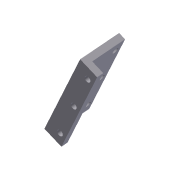
# Autodesk Inventor part: Trapezium
Saved by Autodesk Inventor 2011 (Build 150239000, 239)
## iProperties
Created: 2010-11-23
Part Number: Trapezium
Document SubType Name: Modeling
Designer: Milton
Density: 2.71 g/cm^3
Mass: 8.52062 g
Surface Area: 26.6037 cm^2
Volume: 3.14414 cm^3
Material: Aluminum-6061
Author: Milton
Autodesk Inventor part; units mm, degrees
ref_plane "YZ Plane" through (0, 0, 0) normal (1, 0, 0) x (0, 1, 0)
ref_plane "XZ Plane" through (0, 0, 0) normal (0, 1, 0) x (-1, 0, 0)
ref_plane "XY Plane" through (0, 0, 0) normal (0, 0, 1) x (1, 0, 0)
ref_plane "Work Plane1" through (-107.0936, 321.7811, -1369.8087) normal (-0.8986472, 0.4364419, 0.044177) x (0.0175477, -0.0648608, 0.99774)
sketch "Sketch2" plane through (-107.0936, 321.7811, -1369.8087) normal (-0.8986472, 0.4364419, 0.044177) x (0.0175477, -0.0648608, 0.99774)
  circle A0 centre (15, 4.5) radius 1.35 projected
  circle A1 centre (15, -12.5) radius 1.35 projected
  circle A2 centre (15, -29.5) radius 1.35 projected
  line L0 (17.8, -32.6) -> (17.8, 6) projected
  line L1 (12.2, -30) -> (12.2, 9) projected
  line L2 (12.2, -34.5) -> (12.2, 9.5)
  circle A3 centre (15, 4.5) radius 1.35
  circle A4 centre (15, -12.5) radius 1.35
  circle A5 centre (15, -29.5) radius 1.35
  line L3 (12.2, 9.5) -> (31.2, 9.5)
  line L4 (12.2, -34.5) -> (31.2, -34.5)
  line L5 (31.2, 6) -> (31.2, -32.6) projected
  line L6 (31.2, -32.6) -> (35.7, -32.6) projected
  line L7 (35.7, -31.975) -> (35.7, -32.6) projected
  line L8 (33.7, -31.975) -> (35.7, -31.975) projected
  line L9 (33.7, -27.025) -> (33.7, -31.975) projected
  line L10 (35.7, -27.025) -> (33.7, -27.025) projected
  line L11 (35.7, -25.525) -> (35.7, -27.025) projected
  line L12 (33.2, -25.525) -> (35.7, -25.525) projected
  line L13 (33.2, -16.475) -> (33.2, -25.525) projected
  line L14 (35.7, -16.475) -> (33.2, -16.475) projected
  line L15 (35.7, -14.975) -> (35.7, -16.475) projected
  line L16 (33.7, -14.975) -> (35.7, -14.975) projected
  line L17 (33.7, -10.025) -> (33.7, -14.975) projected
  line L18 (35.7, -10.025) -> (33.7, -10.025) projected
  line L19 (35.7, -8.525) -> (35.7, -10.025) projected
  line L20 (33.2, -8.525) -> (35.7, -8.525) projected
  line L21 (33.2, 0.525) -> (33.2, -8.525) projected
  line L22 (35.7, 0.525) -> (33.2, 0.525) projected
  line L23 (35.7, 2.025) -> (35.7, 0.525) projected
  line L24 (33.7, 2.025) -> (35.7, 2.025) projected
  line L25 (33.7, 6) -> (33.7, 2.025) projected
  line L26 (33.7, 6) -> (31.2, 6) projected
  line L27 (31.2, 9.5) -> (31.2, -34.5)
  line L28 (28.2, 9.5) -> (28.2, -34.5)
  dimension "d1" = 2.7
  dimension "d2" = 2.7
  dimension "d3" = 2.7
  dimension "d6" = 5
  dimension "d8" = 5
  dimension "d13" = 3
  constraints: 10 end point, 3 centre point, 3 coincident, 2 point on line, 1 collinear, 1 parallel, 1 perpendicular
  measures "d1" diameter of A3
  measures "d2" diameter of A4
  measures "d3" diameter of A5
  measures "d6" distance from line of L3 A0.centre
  measures "d8" distance from line of L4 A2.centre
  measures "d13" distance between parallel lines of L5 L28
extrude "Extrusion2" add sketch "Sketch2" along normal blind 3 contours L1 L2 L3 L28 L4 | L28 L3 L27 L5 L4
sketch "Sketch3" plane through (-107.0936, 321.7811, -1369.8087) normal (0.8986472, -0.4364419, -0.044177) x (-0.0175477, 0.0648608, -0.99774)
  circle A0 centre (-15, 4.5) radius 1.35 projected
  circle A1 centre (-15, -29.5) radius 1.35 projected
  circle A2 centre (-15, -12.5) radius 1.35 projected
  line L0 (-31.2, -34.5) -> (-31.2, 9.5) projected
  line L1 (-12.2, -34.5) -> (-31.2, -34.5) projected
  line L2 (-12.2, 9.5) -> (-12.2, -34.5) projected
  line L3 (-31.2, 9.5) -> (-12.2, 9.5) projected
  point P0 (-1389.4632, -172.471)
sketch "Sketch4" plane through (-109.7896, 323.0904, -1369.6761) normal (-0.8986472, 0.4364419, 0.044177) x (0.0175477, -0.0648608, 0.99774)
  line L0 (12.2, -34.5) -> (31.2, -34.5) projected
  line L1 (31.2, 9.5) -> (28.2, 9.5)
  line L2 (28.2, 9.5) -> (28.2, -34.5)
  line L3 (28.2, -34.5) -> (31.2, -34.5)
  line L4 (31.2, -34.5) -> (31.2, 9.5)
  dimension "d16" = 3
  constraints: 8 end point, 2 parallel, 1 horizontal, 1 perpendicular, 1 point on line
  measures "d16" distance of L3.end L2.end
ref_plane "Work Plane2" through (-113.4024, 293.0987, -1341.5395) normal (-0.8986472, 0.4364419, 0.044177) x (0.0175477, -0.0648608, 0.99774)
extrude "Extrusion3" add sketch "Sketch4" against normal up to surface (8.6 mm away)
sketch "Sketch5" plane through (-121.7209, 288.992, -1343.4191) normal (-0.0175477, 0.0648608, -0.99774) x (-0.8986472, 0.4364419, 0.044177)
  circle A0 centre (-2.8, 39) radius 1.35 projected
  circle A1 centre (-2.8, 22) radius 1.35 projected
  circle A2 centre (-2.8, 5) radius 1.35 projected
  circle A3 centre (-2.8, 5) radius 1.35
  circle A4 centre (-2.8, 22) radius 1.35
  circle A5 centre (-2.8, 39) radius 1.35
  point P0 (-176.1642, -137.971)
  dimension "d19" = 2.7
  dimension "d20" = 2.7
  dimension "d21" = 2.7
  constraints: 3 centre point, 3 coincident
  measures "d19" diameter of A3
  measures "d20" diameter of A4
  measures "d21" diameter of A5
extrude "Extrusion4" cut sketch "Sketch5" against normal through all
body "Solid2"
